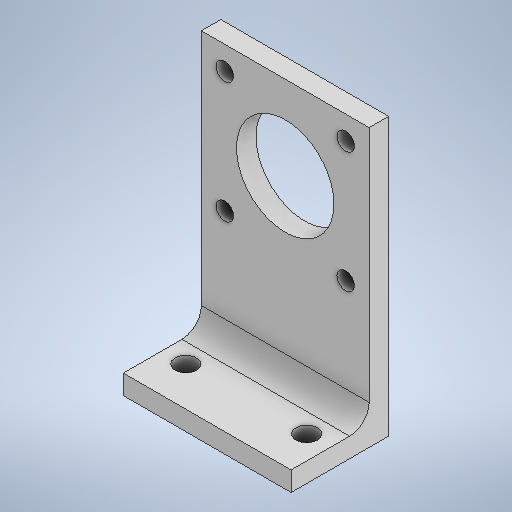
# Autodesk Inventor part: motor_holder
Saved by Autodesk Inventor 2025 (Build 290162010, 162A)
## iProperties
Created: 2025-01-16
Part Number: motor_holder
Material: Generic
Document SubType Name: Modeling
Designer: aduwa
Density: 1 g/cm^3
Appearance: Default
Author: aduwa
Autodesk Inventor part; units mm, degrees
ref_plane "YZ Plane" through (0, 0, 0) normal (1, 0, 0) x (0, 1, 0)
ref_plane "XZ Plane" through (0, 0, 0) normal (0, 1, 0) x (-1, 0, 0)
ref_plane "XY Plane" through (0, 0, 0) normal (0, 0, 1) x (1, 0, 0)
sketch "Sketch1" plane through (0, 0, 0) normal (0, 0, 1) x (1, 0, 0)
  circle A0 centre (0, 0) radius 2.25
  circle A1 centre (31, 0) radius 2.25
  circle A2 centre (0, 31) radius 2.25
  circle A3 centre (31, 31) radius 2.25
  circle A4 centre (15.5, 15.5) radius 12.5
  line L0 (-6, 37) -> (37, 37)
  line L1 (37, 37) -> (37, -6)
  line L2 (37, -6) -> (-6, -6)
  line L3 (-6, -6) -> (-6, 37)
  line L4 (-6, 37) -> (37, -6) construction
  line L5 (37, 37) -> (-6, -6) construction
  line L6 (-6, -6) -> (37, -6)
  line L7 (37, -6) -> (37, -34)
  line L8 (37, -34) -> (-6, -34)
  line L9 (-6, -34) -> (-6, -6)
  dimension "d3" = 4.5
  dimension "d5" = 31
  dimension "d6" = 25
  dimension "d7" = 43
  dimension "d8" = 43
  dimension "d9" = 49.5
  dimension "d10" = 31
  constraints: 20 end point, 5 centre point, 4 parallel, 3 equal radius, 2 horizontal, 2 midpoint, 2 perpendicular, 2 vertical alignment, 1 horizontal alignment
  measures "d3" diameter of A0
  measures "d5" distance of A0.centre A2.centre
  measures "d6" diameter of A4
  measures "d7" distance of L1.end L2.end
  measures "d8" distance of L0.end L1.end
  measures "d9" distance from line of L8 A4.centre
  measures "d10" distance of A3.centre A2.centre
extrude "Extrusion1" add sketch "Sketch1" against normal blind 5
sketch "Sketch2" plane through (0, 0, 0) normal (0, 0, 1) x (1, 0, 0)
  line L0 (37, -34) -> (-6, -34) projected
  line L1 (37, 37) -> (37, -34) projected
  line L2 (-6, -34) -> (37, -34)
  line L3 (37, -34) -> (37, -29)
  line L4 (37, -29) -> (-6, -29)
  line L5 (-6, -29) -> (-6, -34)
  point P0 (0, 0)
  dimension "d13" = 5
  constraints: 8 end point, 2 parallel, 1 horizontal, 1 perpendicular, 1 point on line
  measures "d13" distance of L3.end L2.end
extrude "Extrusion2" add sketch "Sketch2" along normal blind 25
sketch "Sketch3" plane through (-6, -29, 0) normal (0, 1, 0) x (1, 0, 0)
  circle A0 centre (6, -10) radius 2.75
  circle A1 centre (37, -10) radius 2.75
  line L0 (0, 5) -> (0, -25) projected
  line L1 (0, 0) -> (0, -25) projected
  line L2 (43, 0) -> (43, -25) projected
  line L3 (0, 5) -> (43, 5) projected
  point P0 (6, 0)
  point P1 (0, -10)
  point P2 (0, -12.5)
  dimension "d16" = 5.5
  dimension "d17" = 31
  dimension "d23" = 6
  dimension "d24" = 15
  constraints: 2 centre point, 2 horizontal alignment, 2 midpoint, 1 equal radius
  measures "d16" diameter of A0
  measures "d17" distance of A1.centre A0.centre
  measures "d23" distance from line of L0 A0.centre
  measures "d24" distance from line of L3 A0.centre
extrude "Extrusion3" cut sketch "Sketch3" against normal blind 25
fillet "Fillet1" radius 5 1 edges at (15.5, -29, 0)
sketch "Sketch4" plane through (-6, -29, 25) normal (0, 1, 0) x (1, 0, 0)
  line L0 (0, 30) -> (0, 0) projected
  line L1 (0, 5) -> (43.1457, 5)
  circle A0 centre (6, 15) radius 2.75 projected
  line L2 (0, 20) -> (43, 20) projected
  line L3 (0, 20) -> (0, 0) projected
  line L4 (43, 0) -> (0, 0) projected
  line L5 (43, 20) -> (43, 0) projected
  circle A1 centre (6, 15) radius 2.75 projected
  circle A2 centre (37, 15) radius 2.75 projected
  point P0 (6, 25)
  point P1 (43, 5)
  dimension "d25" = 10
  constraints: 2 end point, 1 perpendicular, 1 point on line
  measures "d25" distance from line of L1 A0.centre
extrude "Extrusion4" cut sketch "Sketch4" against normal through all contours L1 L5 L4 L0
body "Solid1"
